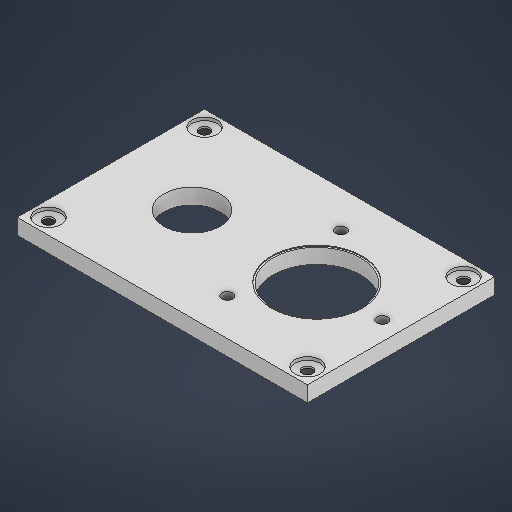
# Autodesk Inventor part: plate
Saved by Autodesk Inventor 2025.2 (Build 292293000, 293)
## iProperties
Created: 2025-04-19
Part Number: plate
Material: Generic
Document SubType Name: Modeling
Designer: klawy
Density: 1 g/cm^3
Appearance: Default
Author: klawy
Autodesk Inventor part; units mm, degrees
ref_plane "YZ Plane" through (0, 0, 0) normal (1, 0, 0) x (0, 1, 0)
ref_plane "XZ Plane" through (0, 0, 0) normal (0, 1, 0) x (-1, 0, 0)
ref_plane "XY Plane" through (0, 0, 0) normal (0, 0, 1) x (1, 0, 0)
sketch "Sketch1" plane through (0, 0, 0) normal (0, 1, 0) x (-1, 0, 0)
  line L0 (46.5, 30) -> (-46.5, 30)
  line L1 (-46.5, 30) -> (-46.5, -30)
  line L2 (-46.5, -30) -> (46.5, -30)
  line L3 (46.5, -30) -> (46.5, 30)
  line L4 (46.5, 30) -> (-46.5, -30) construction
  line L5 (-46.5, 30) -> (46.5, -30) construction
  circle A0 centre (20.5, 0) radius 9
  circle A1 centre (-19.5, 0) radius 12.5
  line L6 (152.1746, 0) -> (-152.1746, 0) construction
  line L7 (0, 58.0523) -> (0, -58.0523) construction
  point P0 (0, 0)
  dimension "d0" = 93
  dimension "d1" = 18
  dimension "d2" = 25
  dimension "d3" = 26
  dimension "d4" = 60
  dimension "d5" = 27
  constraints: 16 end point, 4 midpoint, 2 centre point, 2 horizontal, 2 parallel, 2 point on line, 1 perpendicular, 1 vertical
  measures "d0" distance of L1.end L2.end
  measures "d1" diameter of A0
  measures "d2" diameter of A1
  measures "d3" distance from line of L3 A0.centre
  measures "d4" distance of L0.end L1.end
  measures "d5" distance from line of L1 A1.centre
extrude "Extrusion1" add sketch "Sketch1" along normal blind 5
sketch "Sketch2" plane through (0, 0, 0) normal (0, -1, 0) x (1, 0, 0)
  line L0 (41.5, 25) -> (-41.5, 25) construction
  line L1 (-41.5, 25) -> (-41.5, -25) construction
  line L2 (-41.5, -25) -> (41.5, -25) construction
  line L3 (41.5, -25) -> (41.5, 25) construction
  line L4 (41.5, 25) -> (-41.5, -25) construction
  line L5 (-41.5, 25) -> (41.5, -25) construction
  line L6 (46.5, -30) -> (-46.5, -30) construction
  line L7 (-46.5, -30) -> (-46.5, 30) construction
  point P0 (0, 0)
  dimension "d11" = 5
  dimension "d12" = 5
  constraints: 12 end point, 4 coincident, 2 midpoint, 2 parallel, 1 horizontal, 1 perpendicular
  measures "d11" distance between parallel lines of L6 L2
  measures "d12" distance between parallel lines of L7 L1
hole "Hole1" at (41.5, 0, -25) at (-41.5, 0, -25) at (-41.5, 0, 25) at (41.5, 0, 25) direction (0, 1, 0) diameter 3.4 end through all counterbore diameter 6.5 counterbore depth 3.4 clearance for "Socket Head Cap Screw ISO 4762" size "M3" standard "ISO"
sketch "Sketch3" plane through (0, 5, 0) normal (0, 1, 0) x (1, 0, 0)
  circle A0 centre (-41.5, 25) radius 1.7 projected
  circle A1 centre (-41.5, 25) radius 4
  circle A2 centre (41.5, -25) radius 1.7 projected
  circle A3 centre (-41.5, -25) radius 1.7 projected
  circle A4 centre (-41.5, 25) radius 1.7 projected
  circle A5 centre (41.5, 25) radius 1.7 projected
  line L0 (46.5, -30) -> (46.5, 30) projected
  line L1 (46.5, 30) -> (-46.5, 30) projected
  line L2 (-46.5, 30) -> (-46.5, -30) projected
  line L3 (-46.5, -30) -> (46.5, -30) projected
  circle A6 centre (41.5, 25) radius 4
  circle A7 centre (-41.5, -25) radius 4
  circle A8 centre (41.5, -25) radius 4
  point P0 (0, 0)
  dimension "d22" = 83
  dimension "d25" = 50
  dimension "d28" = 8
  constraints: 4 centre point, 1 coincident, 1 horizontal, 1 vertical, 6 other
  measures "d22" distance of A1.centre A6.centre
  measures "d25" distance of A1.centre A7.centre
  measures "d28" diameter of A1
extrude "Extrusion2" cut sketch "Sketch3" against normal blind 1 contours A0 | A1 | A2 | A3 | A5 | A6 | A7 | A8
sketch "Sketch4" plane through (0, 5, 0) normal (0, 1, 0) x (1, 0, 0)
  circle A0 centre (41.5, -25) radius 4 projected
  circle A1 centre (41.5, 25) radius 4 projected
  circle A2 centre (-41.5, -25) radius 4 projected
  circle A3 centre (-41.5, 25) radius 4 projected
  line L0 (46.5, -30) -> (46.5, 30) projected
  line L1 (46.5, 30) -> (-46.5, 30) projected
  line L2 (-46.5, 30) -> (-46.5, -30) projected
  line L3 (-46.5, -30) -> (46.5, -30) projected
  circle A4 centre (-20.5, 0) radius 9 projected
  circle A5 centre (19.5, 0) radius 12.5 projected
  circle A6 centre (19.5, 0) radius 14
  point P0 (0, 0)
  dimension "d31" = 28
  constraints: 1 centre point, 1 coincident
  measures "d31" diameter of A6
extrude "Extrusion3" cut sketch "Sketch4" against normal through all contours A6
sketch "Sketch6" plane through (0, 5, 0) normal (0, 1, 0) x (1, 0, 0)
  circle A0 centre (19.5, 0) radius 14 projected
  circle A1 centre (19.5, 0) radius 21 construction
  line L0 (-65.1, 0) -> (65.1, 0) projected
  line L1 (19.5, 0) -> (9, -18.1865) construction
  point P0 (40.5, 0)
  point P1 (9, 18.1865)
  dimension "d40" = 42
  dimension "d43" = 360
  dimension "d66" = 60
  constraints: 2 end point, 1 coincident, 1 horizontal alignment, 6 other
  measures "d66" angle of L1 L0
hole "Hole2" at (40.5, 5, 0) at (9, 5, -18.1865) at (9, 5, 18.1865) direction (0, -1, 0) diameter 3.4 end through all clearance for "Socket Head Cap Screw ISO 4762" size "M3" standard "ISO"
sketch "Sketch9" plane through (0, 0, 0) normal (0, -1, 0) x (1, 0, 0)
  circle A0 centre (19.5, 0) radius 12.5 projected
  circle A1 centre (19.5, 0) radius 21 construction
  line L0 (-65.1, 0) -> (65.1, 0) projected
  line L1 (-1.5, 0) -> (19.5, 0) construction
  point P0 (0, 0)
  point P1 (30, 18.1865)
  point P2 (30, -18.1865)
  dimension "d53" = 42
  dimension "d63" = 360
  constraints: 2 end point, 1 coincident, 1 collinear, 7 other
hole "Hole3" at (30, 0, 18.1865) at (30, 0, -18.1865) direction (0, 1, 0) diameter 3 depth 4 tip angle 120
sketch "Sketch10" plane through (0, 5, 0) normal (0, 1, 0) x (1, 0, 0)
  circle A0 centre (19.5, 0) radius 14 projected
  circle A1 centre (19.5, 0) radius 14.5
  point P0 (0, 0)
  dimension "d70" = 0.5
  constraints: 1 centre point, 1 coincident
  measures "d70" radial gap between concentric circles of A0 A1
extrude "Extrusion5" cut sketch "Sketch10" against normal blind 0.25
body "Solid1"
